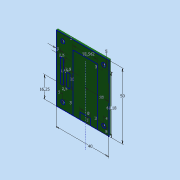
# Autodesk Inventor part: Motherboard_dummy
Saved by Autodesk Inventor 2015 (Build 190159000, 159)
## iProperties
Created: 2014-12-25
Part Number: Motherboard_dummy
Material: ABS Plastic
Document SubType Name: Modeling
Designer: Openlab
Density: 1.06 g/cm^3
Appearance: Smooth - Dark Forest Green
Author: Openlab
Autodesk Inventor part; units mm, degrees
ref_plane "YZ Plane" through (0, 0, 0) normal (1, 0, 0) x (0, 1, 0)
ref_plane "XZ Plane" through (0, 0, 0) normal (0, 1, 0) x (-1, 0, 0)
ref_plane "XY Plane" through (0, 0, 0) normal (0, 0, 1) x (1, 0, 0)
sketch "Sketch1" plane through (0, 0, 0) normal (0, 1, 0) x (-1, 0, 0)
  line L0 (0, 0) -> (0, 50)
  line L1 (40, 50) -> (40, 0)
  line L2 (40, 0) -> (0, 0)
  line L3 (0, 50) -> (40, 50)
  line L4 (27.271, 0) -> (8.729, 0)
  line L5 (8.729, 0) -> (8.729, 43.18)
  line L6 (8.729, 43.18) -> (27.271, 43.18)
  line L7 (27.271, 43.18) -> (27.271, 0)
  line L8 (18, -18.3373) -> (18, 40.4461) construction
  line L9 (14, 5) -> (22, 5)
  line L10 (22, 5) -> (22, 0)
  line L11 (22, 0) -> (14, 0)
  line L12 (14, 0) -> (14, 5)
  circle A0 centre (35, 45) radius 1.5
  circle A1 centre (4, 45) radius 1.5
  circle A2 centre (35, 5) radius 1.5
  circle A3 centre (4, 5) radius 1.5
  line L13 (34.5, 16.25) -> (34.5, 33.75)
  line L14 (34.5, 33.75) -> (37, 33.75)
  line L15 (37, 33.75) -> (37, 16.25)
  line L16 (37, 16.25) -> (34.5, 16.25)
  line L17 (29.5, 16.25) -> (29.5, 26.25)
  line L18 (29.5, 26.25) -> (32, 26.25)
  line L19 (32, 26.25) -> (32, 16.25)
  line L20 (32, 16.25) -> (29.5, 16.25)
  dimension "d42" = 5
  dimension "d43" = 5
  dimension "d44" = 4
  dimension "d45" = 5
  dimension "d47" = 18.542
  dimension "d48" = 18
  dimension "d49" = 43.18
  dimension "d50" = 5
  dimension "d51" = 8
  dimension "d52" = 40
  dimension "d53" = 50
  dimension "d54" = 3
  dimension "d55" = 3
  dimension "d56" = 3
  dimension "d57" = 3
  dimension "d58" = 16.25
  dimension "d59" = 2.5
  dimension "d60" = 2.5
  dimension "d61" = 10
  dimension "d62" = 17.5
  dimension "d63" = 3
  dimension "d64" = 2.5
  constraints: 42 end point, 11 perpendicular, 8 coincident, 4 centre point, 3 collinear, 3 horizontal alignment, 2 vertical alignment, 2 other
  measures "d42" distance from line of L3 A1.centre
  measures "d43" distance from line of L2 A3.centre
  measures "d44" distance from line of L0 A3.centre
  measures "d45" distance from line of L1 A2.centre
  measures "d47" distance of L6.start L6.end
  measures "d48" distance between parallel lines of L8 L0
  measures "d49" distance of L4.end L6.start
  measures "d50" distance of L11.end L9.start
  measures "d51" distance of L9.start L9.end
  measures "d52" distance of L2.start L2.end
  measures "d53" distance of L2.end L3.start
  measures "d54" diameter of A3
  measures "d55" diameter of A1
  measures "d56" diameter of A2
  measures "d57" diameter of A0
  measures "d58" distance between parallel lines of L2 L20
  measures "d59" distance of L14.start L14.end
  measures "d60" distance of L18.start L18.end
  measures "d61" distance of L17.start L18.start
  measures "d62" distance of L13.start L14.start
  measures "d63" distance between parallel lines of L1 L15
  measures "d64" distance between parallel lines of L13 L19
extrude "Extrusion1" add sketch "Sketch1" along normal blind 1.5 contours L0 L3 L1 L2 L7 L6 L5 | L5 L6 L7 L2 L10 L9 L12 | L12 L9 L10 L2 | L13 L14 L15 L16 | L17 L18 L19 L20
extrude "Extrusion2" add sketch "Sketch1" along normal blind 5 contours L5 L6 L7 L2 L10 L9 L12 | L12 L9 L10 L2
extrude "Extrusion3" add sketch "Sketch1" along normal blind 7 contours L12 L9 L10 L2
extrude "Extrusion4" add sketch "Sketch1" along normal blind 10 contours L13 L14 L15 L16 | L17 L18 L19 L20
body "Solid1"
